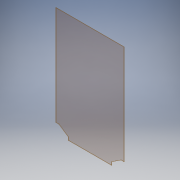
# Autodesk Inventor part: Belly_pan
Saved by Autodesk Inventor 2018 (Build 220112000, 112)
## iProperties
Created: 2018-09-06
Part Number: Belly_pan
Material: Generic
Document SubType Name: Modeling
Designer: baoan
Density: 1 g/cm^3
Appearance: Polycarbonate - Smoked
Author: baoan
Autodesk Inventor part; units mm, degrees
ref_plane "YZ Plane" through (0, 0, 0) normal (1, 0, 0) x (0, 1, 0)
ref_plane "XZ Plane" through (0, 0, 0) normal (0, 1, 0) x (-1, 0, 0)
ref_plane "XY Plane" through (0, 0, 0) normal (0, 0, 1) x (1, 0, 0)
sketch "Sketch1" plane through (0, 0, 0) normal (0, 0, 1) x (1, 0, 0)
  line L0 (-254, -431.8) -> (-177.8, -431.8) construction
  line L1 (254, -431.8) -> (254, -381) construction
  line L2 (254, 431.8) -> (-254, 431.8)
  line L3 (-254, 431.8) -> (-254, -381) construction
  line L4 (-254, -431.8) -> (254, 431.8) construction
  line L5 (254, -431.8) -> (-254, 431.8) construction
  line L6 (-254, -381) -> (-177.8, -431.8)
  line L7 (177.8, -431.8) -> (254, -381)
  line L8 (-254, -381) -> (-254, -431.8) construction
  line L9 (-177.8, -431.8) -> (177.8, -431.8) construction
  line L10 (177.8, -431.8) -> (254, -431.8) construction
  line L11 (254, -381) -> (254, 431.8) construction
  line L12 (-254, 431.8) -> (-279.4, 431.8)
  line L13 (-279.4, 431.8) -> (-279.4, -381)
  line L14 (-254, -381) -> (-279.4, -381)
  line L15 (279.4, 431.8) -> (279.4, -381)
  line L16 (279.4, 431.8) -> (254, 431.8)
  line L17 (279.4, -381) -> (254, -381)
  line L18 (-177.8, -431.8) -> (-177.8, -457.2)
  line L19 (-177.8, -457.2) -> (177.8, -457.2)
  line L20 (177.8, -457.2) -> (177.8, -431.8)
  point P0 (0, 0)
  dimension "d0" = 508
  dimension "d1" = 863.6
  dimension "d2" = 50.8
  dimension "d3" = 76.2
  dimension "d4" = 76.2
  dimension "d5" = 50.8
  dimension "d8" = 25.4
  dimension "d9" = 812.8
  dimension "d10" = 812.8
  dimension "d11" = 25.4
  dimension "d12" = 25.4
  dimension "d13" = 355.6
  constraints: 42 end point, 8 perpendicular, 7 parallel, 6 horizontal, 2 midpoint, 1 point on line, 1 vertical
  measures "d0" distance of L2.start L2.end
  measures "d1" distance of L2.start L1.start
  measures "d2" distance of L1.end L1.start
  measures "d3" distance of L1.start L7.start
  measures "d4" distance of L0.start L0.end
  measures "d5" distance of L0.start L3.end
  measures "d8" distance of L2.end L12.end
  measures "d9" distance of L12.end L13.end
  measures "d10" distance of L15.start L15.end
  measures "d11" distance of L15.start L2.start
  measures "d12" distance of L0.end L18.end
  measures "d13" distance of L18.end L19.end
extrude "Extrusion1" add sketch "Sketch1" along normal mid plane 3.175
equation "\"d4\" = d3"
equation "\"d5\" = d2"
body "Solid1"
